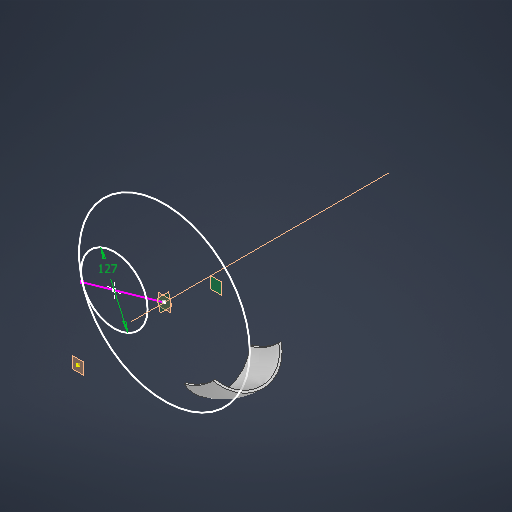
# Autodesk Inventor part: подьем колеса 25-26
Saved by Autodesk Inventor 2025 (Build 290162000, 162)
## iProperties
Created: 2025-10-03
Part Number: подьем колеса 25-26
Material: Типовые
Document SubType Name: Modeling
Designer: Phantom
Density: 1 g/cm^3
Appearance: По умолчанию
Author: Phantom
Autodesk Inventor part; units mm, degrees
ref_plane "YZ Plane" through (0, 0, 0) normal (1, 0, 0) x (0, 1, 0)
ref_plane "XZ Plane" through (0, 0, 0) normal (0, 1, 0) x (-1, 0, 0)
ref_plane "XY Plane" through (0, 0, 0) normal (0, 0, 1) x (1, 0, 0)
ref_plane "РабПлоскость15" through (0, 0, 121) normal (0, 0, -1) x (-1, 0, 0)
ref_plane "РабПлоскость11" through (0, 0, 385) normal (0, 0, 1) x (1, 0, 0)
ref_plane "РабПлоскость2" through (165.364, 186.5392, 385) normal (-0.9611557, -0.2760066, 0) x (0.2760066, -0.9611557, 0)
ref_plane "РабПлоскость3" through (165.364, 186.5392, 385) normal (0, 0, 1) x (1, 0, 0)
sketch "Эскиз18" plane through (165.364, 186.5392, 385) normal (0, 0, 1) x (1, 0, 0)
  circle A0 centre (0, 0) radius 163
  line L0 (0, 0) -> (-156.6684, -44.9891) projected
  circle A1 centre (-95.635, -27.4627) radius 63.5
  point P0 (-165.364, -186.5392)
  dimension "d55" = 127
  constraints: 1 centre point, 1 coincident, 1 point on line, 3 other
  measures "d55" diameter of A1
ref_plane "РабПлоскость6" through (8.6956, 141.5501, 121) normal (-0.3087313, -0.9511493, 0) x (0.9511493, -0.3087313, 0)
ref_plane "РабПлоскость14" through (0, 0, 121) normal (0, 0, -1) x (-1, 0, 0)
ref_plane "РабПлоскость16" through (0, 0, 385) normal (0, 0, 1) x (1, 0, 0)
sketch "Эскиз43" plane through (165.364, 186.5392, 385) normal (-0.9611557, -0.2760066, 0) x (0.2760066, -0.9611557, 0)
  line L0 (163, 0) -> (-163, 0) projected
  circle A0 centre (96.5, -68.2373) radius 66.5
  circle A1 centre (96.5, -68.2373) radius 70.5
  line L1 (124.2095, 7.1873) -> (124.2095, -174.1782)
  line L2 (0, -463.4375) -> (0, 85.6248) projected
  point P0 (133.6516, -385)
  point P1 (124.2095, -3.4111)
  point P2 (124.2095, -7.7854)
  point P3 (124.2095, -128.6892)
  point P4 (124.2095, -133.0634)
  dimension "d140" = 133
  dimension "d141" = 141
  dimension "d144" = 96.5
  constraints: 2 centre point, 2 end point, 1 coincident, 1 vertical
  measures "d140" diameter of A0
  measures "d141" diameter of A1
  measures "d144" distance from line of L2 A0.centre
revolve "Вращение3" add sketch "Эскиз43" angle 30 about axis through (165.364, 186.5392, 385) along (0, 0, 1) contours A1 L1 A0
